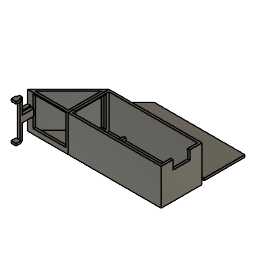
FirstPrototype (Autodesk Fusion 360 design; units mm, degrees)
part number: 2026-07-30-17-18-59-911
part number: 2026-07-30-18-52-39-919
part number: 2026-07-30-22-07-18-426
part number: 2026-07-30-22-07-47-172
part number: 2026-07-31-14-05-23-985
part number: 2026-08-03-20-47-02-403
Autodesk Fusion 360 part; units mm, degrees
note: some values were not read from the file. Set by a fixed rule: which sketch regions a step uses.
sketch "Sketch1" plane through (0, 0, 0) normal (0, 1, 0) x (1, 0, 0) in component "Display_Lens"
sketch "Sketch2" plane through (0, 0, 0) normal (0, 0, 1) x (1, 0, 0) in component "Display_Lens"
  line L0 (0, 0) -> (82, 0)
  line L1 (82, 0) -> (82, 36)
  line L2 (82, 36) -> (0, 36)
  line L3 (0, 36) -> (0, 0)
  dimension "d1" = 82
  dimension "d2" = 36
  constraint horizontal L0
  constraint vertical L1
  constraint horizontal L2
  constraint vertical L3
  constraint coincident L0.start L3.end
  measures "d1" distance of L0.start L0.end
  measures "d2" distance of L0.start L2.end
extrude "ExtrudedCentralBase" add sketch "Sketch2" along normal blind 34 makes body 1 in component "Display_Lens"
shell "Removed2mmTop" thickness 2 removed faces 1 at (27.3333, 24, 34) on bodies 1 in component "Display_Lens"
sketch "CreatedLensViewWindow" plane through (2, 0, 0) normal (1, 0, 0) x (0, 1, 0) in component "Display_Lens"
  line L0 (2, 2) -> (34, 2)
  line L1 (34, 2) -> (34, 34)
  line L2 (34, 34) -> (2, 34)
  line L3 (2, 34) -> (2, 2)
  line L4 (4.5, 31.5) -> (31.5, 31.5)
  line L5 (31.5, 31.5) -> (31.5, 4.5)
  line L6 (31.5, 4.5) -> (4.5, 4.5)
  line L7 (4.5, 4.5) -> (4.5, 31.5)
  line L8 (4.5, 31.5) -> (31.5, 4.5) construction
  line L9 (31.5, 31.5) -> (4.5, 4.5) construction
  point P0 (18, 18)
  dimension "d8" = 27
  dimension "d9" = 27
  constraint horizontal L4
  constraint perpendicular L4 L5
  constraint parallel L4 L6
  constraint parallel L5 L7
  constraint coincident L8 P0
  constraint coincident L9 P0
  measures "d8" distance of L5.end L6.end
  measures "d9" distance of L4.end L5.end
extrude "ExtrudeOledViewWindow" cut sketch "CreatedLensViewWindow" against normal blind 2 contours L4 L5 L6 L7 bodies 1 in component "Display_Lens"
sketch "CreatedOledBackHold" plane through (0, 0, 2) normal (0, 0, 1) x (-1, 0, 0) in component "Display_Lens"
  line L0 (-2, -34) -> (-2, -2)
  line L1 (-2, -2) -> (-80, -2)
  line L2 (-80, -2) -> (-80, -34)
  line L3 (-80, -34) -> (-2, -34)
  line L4 (-17, -2) -> (-15, -2)
  line L5 (-15, -2) -> (-15, -34)
  line L6 (-15, -34) -> (-17, -34)
  line L7 (-17, -34) -> (-17, -2)
  constraint horizontal L4
  constraint vertical L5
  constraint horizontal L6
  constraint vertical L7
  constraint coincident L3 L5.end
  constraint coincident L1 L4.start
extrude "ExtrudeOledBackHold" add sketch "CreatedOledBackHold" along normal blind 2.5 contours L1 L3 L4 L5 L6 L7 bodies 1 in component "Display_Lens"
sketch "ConstructCableSpace" plane through (82, 0, 0) normal (1, 0, 0) x (0, 1, 0) in component "Display_Lens"
  line L0 (0, 0) -> (36, 0)
  line L1 (36, 0) -> (36, 34)
  line L2 (36, 34) -> (0, 34)
  line L3 (0, 34) -> (0, 0)
  line L4 (10.5, 34) -> (25.5, 34)
  line L5 (25.5, 34) -> (25.5, 24)
  line L6 (25.5, 24) -> (10.5, 24)
  line L7 (10.5, 24) -> (10.5, 34)
  dimension "d14" = 15
  dimension "d15" = 10
  constraint horizontal L4
  constraint vertical L5
  constraint horizontal L6
  constraint vertical L7
  constraint collinear L2 L4
  measures "d14" distance of L4.start L4.end
  measures "d15" distance of L4.start L6.end
extrude "MadeCableSpace" cut sketch "ConstructCableSpace" against normal blind 2 contours L2 L4 L5 L6 L7 bodies 1 in component "Display_Lens"
extrude "MadeTop2mmSmaller" cut 1 faces at (28, 0.6667, 34) along direction (0, 0, -1) blind 2 on bodies 1 bodies 1 in component "Display_Lens"
sketch "CreateOledHolder" plane through (0, 0, 2) normal (0, 0, 1) x (-1, 0, 0) in component "Display_Lens"
  line L0 (-17, -34) -> (-17, -2)
  line L1 (-17, -2) -> (-80, -2)
  line L2 (-80, -2) -> (-80, -34)
  line L3 (-80, -34) -> (-17, -34)
  line L4 (-77, -28) -> (-75, -28)
  line L5 (-75, -28) -> (-75, -8)
  line L6 (-75, -8) -> (-77, -8)
  line L7 (-77, -8) -> (-77, -28)
  dimension "d23" = 3
  constraint horizontal L4
  constraint vertical L5
  constraint horizontal L6
  constraint vertical L7
  measures "d23" distance of L2 L7
extrude "ExtrudeOledHolder" add sketch "CreateOledHolder" along normal blind 3 contours L4 L5 L6 L7 bodies 1 in component "Display_Lens"
sketch "MadeFirstNotch" plane through (80, 0, 0) normal (-1, 0, 0) x (0, -1, 0) in component "Display_Lens"
  line L0 (-25.5, 32) -> (-34, 32)
  line L1 (-34, 32) -> (-34, 2)
  line L2 (-34, 2) -> (-2, 2)
  line L3 (-2, 2) -> (-2, 32)
  line L4 (-2, 32) -> (-10.5, 32)
  line L5 (-10.5, 32) -> (-10.5, 24)
  line L6 (-10.5, 24) -> (-25.5, 24)
  line L7 (-25.5, 24) -> (-25.5, 32)
  line L8 (-28.8, 28.8) -> (-28, 28.8)
  line L9 (-28, 28.8) -> (-28, 28)
  line L10 (-28, 28) -> (-28.8, 28)
  line L11 (-28.8, 28) -> (-28.8, 28.8)
  dimension "d26" = 0.8
  dimension "d27" = 0.8
  dimension "d29" = 5.2
  dimension "d43" = 3.2
  constraint horizontal L8
  constraint vertical L9
  constraint horizontal L10
  constraint vertical L11
  measures "d26" distance of L8.start L8.end
  measures "d27" distance of L8.start L10.end
  measures "d29" distance of L1 L11
  measures "d43" distance of L0 L8
extrude "ExtrudeFirstNotch" add sketch "MadeFirstNotch" along normal blind 3 contours L8 L9 L10 L11 bodies 1 in component "Display_Lens"
sketch "madeSecondNotch" plane through (80, 0, 0) normal (-1, 0, 0) x (0, -1, 0) in component "Display_Lens"
  line L0 (-28.8, 28) -> (-28.8, 28.8)
  line L1 (-28.8, 28.8) -> (-28, 28.8)
  line L2 (-28, 28.8) -> (-28, 28)
  line L3 (-28, 28) -> (-28.8, 28)
  line L4 (-25.5, 32) -> (-34, 32)
  line L5 (-34, 32) -> (-34, 2)
  line L6 (-34, 2) -> (-2, 2)
  line L7 (-2, 2) -> (-2, 32)
  line L8 (-2, 32) -> (-10.5, 32)
  line L9 (-10.5, 32) -> (-10.5, 24)
  line L10 (-10.5, 24) -> (-25.5, 24)
  line L11 (-25.5, 24) -> (-25.5, 32)
  line L12 (-8, 28.8) -> (-7.2, 28.8)
  line L13 (-7.2, 28.8) -> (-7.2, 28)
  line L14 (-7.2, 28) -> (-8, 28)
  line L15 (-8, 28) -> (-8, 28.8)
  dimension "d32" = 0.8
  dimension "d33" = 0.8
  dimension "d35" = 5.2
  dimension "d42" = 3.2
  constraint horizontal L12
  constraint vertical L13
  constraint horizontal L14
  constraint vertical L15
  measures "d32" distance of L12.start L12.end
  measures "d33" distance of L12.start L14.end
  measures "d35" distance of L7 L13
  measures "d42" distance of L8 L12
extrude "ExtrudeSecondNotch" add sketch "madeSecondNotch" along normal blind 3 contours L12 L13 L14 L15 bodies 1 in component "Display_Lens"
sketch "CreatedMirrorTriangle" plane through (0, 0, 0) normal (0, 0, 1) x (1, 0, 0) in component "MirrorModule"
  line L0 (0, 36) -> (0, 0)
  line L1 (0, 36) -> (0, 0)
  line L2 (0, 0) -> (-36, 0)
  line L3 (-36, 0) -> (0, 36)
  dimension "d53" = 50.9117
  dimension "d54" = 36
  constraint coincident L0.end L1.end
  constraint vertical L0
  constraint perpendicular L1 L2
  measures "d53" distance of L0.start L2.end
  measures "d54" distance of L0 L2.end
extrude "Extrude1" add sketch "CreatedMirrorTriangle" along normal blind 32 separate body makes body 2 in component "MirrorModule"
shell "MadeMirror2mmShell" thickness 2 removed faces 1 at (-12, 12, 32) on bodies 2 in component "MirrorModule"
sketch "FirstMirrorOpeningCreate" plane through (0, 0, 0) normal (1, 0, 0) x (0, 1, 0) in component "MirrorModule"
  line L0 (0, 0) -> (36, 0)
  line L1 (36, 0) -> (36, 32)
  line L2 (36, 32) -> (0, 32)
  line L3 (0, 32) -> (0, 0)
  line L4 (4.4855, 31.4876) -> (31.4855, 31.4876)
  line L5 (31.4855, 31.4876) -> (31.4855, 4.4876)
  line L6 (31.4855, 4.4876) -> (4.4855, 4.4876)
  line L7 (4.4855, 4.4876) -> (4.4855, 31.4876)
  dimension "d55" = 27
  dimension "d56" = 27
  constraint horizontal L4
  constraint vertical L5
  constraint horizontal L6
  constraint vertical L7
  measures "d55" distance of L4.start L4.end
  measures "d56" distance of L4.start L6.end
extrude "ExtrudeFirstMOpenning" cut sketch "FirstMirrorOpeningCreate" against normal blind 2 contours L4 L5 L6 L7 bodies 2 in component "MirrorModule"
sketch "SecondMirrorOp.Created" plane through (0, 0, 0) normal (0, -1, 0) x (1, 0, 0) in component "MirrorModule"
  line L0 (-36, 0) -> (0, 0)
  line L1 (0, 0) -> (0, 32)
  line L2 (0, 32) -> (-36, 32)
  line L3 (-36, 32) -> (-36, 0)
  line L4 (-31, 31) -> (-2.0207, 31)
  line L5 (-2.0207, 31) -> (-2.0207, 4.5)
  line L6 (-2.0207, 4.5) -> (-31, 4.5)
  line L7 (-31, 4.5) -> (-31, 31)
  dimension "d61" = 4.5
  dimension "d62" = 1
  constraint horizontal L4
  constraint vertical L5
  constraint horizontal L6
  constraint vertical L7
  measures "d61" distance of L0 L6
  measures "d62" distance of L2 L4
extrude "SndMirrorOpeningExtruded" cut sketch "SecondMirrorOp.Created" against normal blind 2 contours L4 L5 L6 L7 bodies 2 in component "MirrorModule"
sketch "definedSliderSupport" plane through (0, 0, 0) normal (0, -1, 0) x (1, 0, 0) in component "BeamSplitterModule"
  line L0 (-2.0207, 31) -> (-2.0207, 4.5)
  line L1 (-2.0207, 4.5) -> (-31, 4.5)
  line L2 (-31, 4.5) -> (-31, 31)
  line L3 (-31, 31) -> (-2.0207, 31)
  line L4 (-36, 0) -> (0, 0)
  line L5 (0, 0) -> (0, 32)
  line L6 (0, 32) -> (-36, 32)
  line L7 (-36, 32) -> (-36, 0)
  line L8 (-36, 21) -> (-33, 21)
  line L9 (-33, 21) -> (-33, 13)
  line L10 (-33, 13) -> (-36, 13)
  line L11 (-36, 13) -> (-36, 21)
  dimension "d71" = 13
  constraint horizontal L8
  constraint vertical L9
  constraint horizontal L10
  constraint vertical L11
  constraint coincident L7 L8.start
  measures "d71" distance of L4 L10
extrude "ExtrudeSliderSupport" add sketch "definedSliderSupport" along normal blind 6 separate body contours L7 L8 L9 L10 L11 makes body 3 in component "BeamSplitterModule"
sketch "Sketch5" plane through (-33, 0, 0) normal (1, 0, 0) x (0, 1, 0) in component "BeamSplitterModule"
  line L0 (0, 13) -> (0, 21)
  line L1 (0, 21) -> (-6, 21)
  line L2 (-6, 21) -> (-6, 13)
  line L3 (-6, 13) -> (0, 13)
  line L4 (0, 20) -> (-10, 20)
  line L5 (-10, 20) -> (-10, 14)
  line L6 (-10, 14) -> (0, 14)
  line L7 (0, 14) -> (0, 20)
  dimension "d74" = 10
  dimension "d75" = 6
  dimension "d76" = 1
  constraint horizontal L4
  constraint vertical L5
  constraint horizontal L6
  constraint vertical L7
  constraint coincident L0 L4.start
  measures "d74" distance of L4.start L4.end
  measures "d75" distance of L4.start L6.end
  measures "d76" distance of L3 L6
extrude "Extrude3" add sketch "Sketch5" along normal blind 2.5 contours L0 L2 L4 L6 L7 | L2 L4 L5 L6 bodies 3 in component "BeamSplitterModule"
sketch "Sketch6" plane through (0, -10, 0) normal (0, -1, 0) x (1, 0, 0) in component "BeamSplitterModule"
  line L0 (-33, 20) -> (-33, 14)
  line L1 (-33, 14) -> (-30.5, 14)
  line L2 (-30.5, 14) -> (-30.5, 20)
  line L3 (-30.5, 20) -> (-33, 20)
  line L4 (-33, 34) -> (-30.5, 34)
  line L5 (-30.5, 34) -> (-30.5, 0)
  line L6 (-30.5, 0) -> (-33, 0)
  line L7 (-33, 0) -> (-33, 34)
  dimension "d79" = 2.5
  dimension "d80" = 34
  constraint horizontal L4
  constraint vertical L5
  constraint horizontal L6
  constraint vertical L7
  measures "d79" distance of L4.start L4.end
  measures "d80" distance of L4.start L6.end
extrude "2mmBeam" add sketch "Sketch6" along normal blind 2 bodies 3 in component "BeamSplitterModule"
sketch "firstPert" plane through (0, -12, 0) normal (0, -1, 0) x (1, 0, 0) in component "BeamSplitterModule"
  line L0 (-33, 0) -> (-30.5, 0)
  line L1 (-30.5, 0) -> (-30.5, 34)
  line L2 (-30.5, 34) -> (-33, 34)
  line L3 (-33, 34) -> (-33, 0)
  line L4 (-34, 34) -> (-29.5, 34)
  line L5 (-29.5, 34) -> (-29.5, 32)
  line L6 (-29.5, 32) -> (-34, 32)
  line L7 (-34, 32) -> (-34, 34)
  constraint horizontal L4
  constraint vertical L5
  constraint horizontal L6
  constraint vertical L7
extrude "Extrude1stPert" add sketch "firstPert" along normal blind 4.5 contours L3 L4 L6 L7 | L1 L2 L3 L4 L6 | L1 L4 L5 L6 bodies 3 in component "BeamSplitterModule"
sketch "2ndPert" plane through (0, -12, 0) normal (0, -1, 0) x (1, 0, 0) in component "BeamSplitterModule"
  line L0 (-33, 32) -> (-33, 0)
  line L1 (-33, 0) -> (-30.5, 0)
  line L2 (-30.5, 0) -> (-30.5, 32)
  line L3 (-34, 2) -> (-29.5, 2)
  line L4 (-29.5, 2) -> (-29.5, 0)
  line L5 (-29.5, 0) -> (-34, 0)
  line L6 (-34, 0) -> (-34, 2)
  line L7 (-30.5, 32) -> (-33, 32)
  constraint horizontal L3
  constraint vertical L4
  constraint horizontal L5
  constraint vertical L6
extrude "ExtrudeSndPerm" add sketch "2ndPert" along normal blind 4.5 contours L0 L1 L2 L3 L5 | L0 L3 L5 L6 | L2 L3 L4 L5 bodies 3 in component "BeamSplitterModule"
sketch "Sketch1 (2)" plane through (0, 0, 0) normal (0, 0, 1) x (1, 0, 0) in component "Cover"
  line L0 (80, 40) -> (0, 40)
  line L1 (0, 40) -> (0, 76)
  line L2 (0, 76) -> (80, 76)
  line L3 (80, 76) -> (80, 40)
  dimension "d88" = 36
  constraint horizontal L0
  constraint vertical L1
  constraint horizontal L2
  constraint vertical L3
  measures "d88" distance of L0.start L2.end
extrude "Extrude1'" add sketch "Sketch1 (2)" along normal blind 2 separate body makes body 4 in component "Cover"
sketch "Sketch2 (2)" plane through (0, 0, 0) normal (0, 0, -1) x (1, 0, 0) in component "Cover"
  line L0 (0, -76) -> (80, -76)
  line L1 (80, -76) -> (80, -40)
  line L2 (80, -40) -> (0, -40)
  line L3 (0, -40) -> (0, -76)
  line L4 (0, -40) -> (-36, -40)
  line L5 (0, -40) -> (0, -76)
  line L6 (-36, -40) -> (0, -76)
  dimension "d91" = 36
  constraint coincident L2.end L3.start
  constraint perpendicular L3 L4
  constraint coincident L0.start L3.end
  measures "d91" distance of L2.end L4.end
extrude "Extrude2" add sketch "Sketch2 (2)" against normal blind 2 contours L3 L4 L5 L6 bodies 4 in component "Cover"
component "Display_Lens" placed x (1, 0, 0) y (0, 1, 0) z (0, 0, 1) at (0, 0, 0)
component "MirrorModule" placed x (1, 0, 0) y (0, 1, 0) z (0, 0, 1) at (0, 0, 0)
component "BeamSplitterModule" placed x (1, 0, 0) y (0, 1, 0) z (0, 0, 1) at (0, 0, 0)
component "Cover" placed x (1, 0, 0) y (0, 1, 0) z (0, 0, 1) at (0, 0, 0)
component "Component" placed x (1, 0, 0) y (0, 1, 0) z (0, 0, 1) at (0, 0, 0) in component "Display_Lens"
equation "OledCapsule = 3 mm" comment "3 mm from back inner plane, 20 mm in length, 2mm in width, 3mm height"
equation "SmallNothesOLED = 0.8 mm" comment "0.8X0.8 NOTHES. 5.2 from left side of inner wall, 5.2 considering outer high wall"
equation "DisplayLensDistance = 65 mm" comment "Distance from inner back wall to inner(front) lens holder"
equation "WallsThickness = 2 mm"
equation "LensOpening = 27 mm" comment "27Width27.5Height"
equation "LensHolderOffset = 13 mm" comment "Offset considerign inner front wall and inner holder wall"
